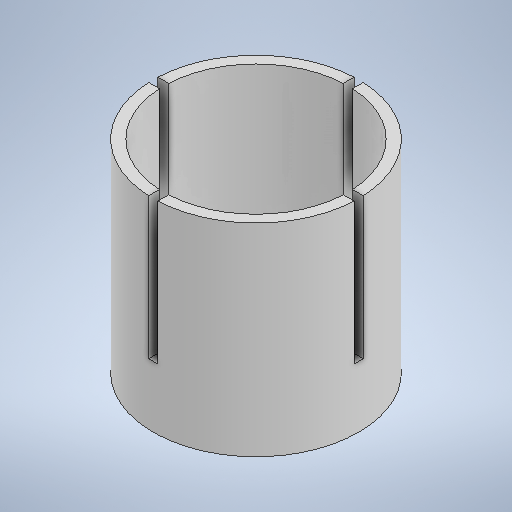
# Autodesk Inventor part: nozzle
Saved by Autodesk Inventor 2025 (Build 290162000, 162)
## iProperties
Created: 2025-03-25
Part Number: nozzle
Material: Generic
Document SubType Name: Modeling
Designer: ethan
Density: 1 g/cm^3
Appearance: Default
Author: ethan
Autodesk Inventor part; units mm, degrees
ref_plane "YZ Plane" through (0, 0, 0) normal (1, 0, 0) x (0, 1, 0)
ref_plane "XZ Plane" through (0, 0, 0) normal (0, 1, 0) x (-1, 0, 0)
ref_plane "XY Plane" through (0, 0, 0) normal (0, 0, 1) x (1, 0, 0)
sketch "Sketch1" plane through (0, 0, 0) normal (0, 1, 0) x (-1, 0, 0)
  circle A0 centre (0, 0) radius 15
  circle A1 centre (0, 0) radius 16.75
  dimension "d0" = 30
  dimension "d1" = 33.5
  constraints: 2 centre point, 2 coincident
  measures "d0" diameter of A0
  measures "d1" diameter of A1
extrude "Extrusion1" add sketch "Sketch1" along normal blind 33
sketch "Sketch2" plane through (0, 33, 0) normal (0, 1, 0) x (1, 0, 0)
  circle A0 centre (0, 0) radius 16.75 construction
  circle A1 centre (0, 0) radius 15 construction
  line L0 (17.6424, -0.75) -> (17.6424, 0.75) construction
  line L1 (17.6424, 0.75) -> (-17.6424, 0.75) construction
  line L2 (-17.6424, 0.75) -> (-17.6424, -0.75) construction
  line L3 (-17.6424, -0.75) -> (17.6424, -0.75) construction
  line L4 (17.6424, -0.75) -> (-17.6424, 0.75) construction
  line L5 (17.6424, 0.75) -> (-17.6424, -0.75) construction
  line L6 (-0.75, -17.7047) -> (-0.75, 17.7047) construction
  line L7 (-0.75, 17.7047) -> (0.75, 17.7047) construction
  line L8 (0.75, 17.7047) -> (0.75, -17.7047) construction
  line L9 (0.75, -17.7047) -> (-0.75, -17.7047) construction
  line L10 (-0.75, -17.7047) -> (0.75, 17.7047) construction
  line L11 (-0.75, 17.7047) -> (0.75, -17.7047) construction
  line L12 (-0.75, -17.7047) -> (0.75, -17.7047)
  line L13 (0.75, -17.7047) -> (0.75, 17.7047)
  line L14 (0.75, 17.7047) -> (-0.75, 17.7047)
  line L15 (-0.75, 17.7047) -> (-0.75, -17.7047)
  line L16 (-17.6424, -0.75) -> (17.6424, -0.75)
  line L17 (17.6424, -0.75) -> (17.6424, 0.75)
  line L18 (17.6424, 0.75) -> (-17.6424, 0.75)
  line L19 (-17.6424, 0.75) -> (-17.6424, -0.75)
  point P0 (-0.75, -0.75)
  point P1 (0.75, -0.75)
  point P2 (0.75, 0.75)
  point P3 (-0.75, 0.75)
  dimension "d4" = 1.5
  dimension "d5" = 1.5
  constraints: 40 end point, 8 parallel, 5 perpendicular, 4 midpoint, 2 horizontal, 1 vertical
  measures "d4" distance of L0.start L0.end
  measures "d5" distance of L6.end L7.end
extrude "Extrusion2" cut sketch "Sketch2" against normal blind 23
body "Solid1"
